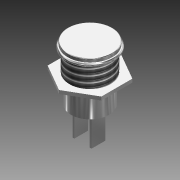
# Autodesk Inventor part: Hohlstecker
Saved by Autodesk Inventor 2013 SP1 (Build 170176100, 176)
## iProperties
Created: 2012-12-09
Part Number: Hohlstecker
Material: Stahl, verchromt
Document SubType Name: Modeling
Designer: Sebastian
Density: 1 g/cm^3
Author: Sebastian
Autodesk Inventor part; units mm, degrees
note: some values were not read from the file. Chosen so that the rebuilt part matches the saved one: edges of "Rundung1".
ref_plane "YZ Plane" through (0, 0, 0) normal (1, 0, 0) x (0, 1, 0)
ref_plane "XZ Plane" through (0, 0, 0) normal (0, 1, 0) x (-1, 0, 0)
ref_plane "XY Plane" through (0, 0, 0) normal (0, 0, 1) x (1, 0, 0)
sketch "Skizze1" plane through (0, 0, 0) normal (0, 0, 1) x (1, 0, 0)
  circle A0 centre (0, 0) radius 5.5
  dimension "d0" = 11
  constraints: 1 centre point, 1 coincident
  measures "d0" diameter of A0
extrude "Extrusion1" add sketch "Skizze1" against normal blind 6
sketch "Skizze2" plane through (0, 0, 0) normal (0, 0, 1) x (1, 0, 0)
  circle A0 centre (0, 0) radius 6
  dimension "d5" = 12
  constraints: 1 centre point, 1 coincident
  measures "d5" diameter of A0
extrude "Extrusion2" add sketch "Skizze2" along normal blind 8 separate body
thread "Gewinde1" size "M12x1.75" class "6g" standard "ANSI Metric M Profile" full length
sketch "Skizze3" plane through (0, 0, 0) normal (0, 0, 1) x (1, 0, 0)
  circle A0 centre (0, 0) radius 5.75
  dimension "d10" = 11.5
  constraints: 1 centre point, 1 coincident
  measures "d10" diameter of A0
extrude "Extrusion3" add sketch "Skizze3" along normal blind 1 separate body
move or copy body "Körper verschieben1" bodies to move or copy 3 copy no translate (0, 0, 8)
fillet "Rundung1" radius 0.5 1 edges at (-6, 0, 0)
sketch "Skizze4" plane through (0, 0, 0) normal (0, 0, 1) x (1, 0, 0)
  circle A0 centre (0, 0) radius 6.5
  dimension "d19" = 13
  constraints: 1 centre point, 1 coincident
  measures "d19" diameter of A0
extrude "Extrusion4" add sketch "Skizze4" along normal blind 1 separate body
move or copy body "Körper verschieben2" bodies to move or copy 4 copy no translate (0, 0, 9)
fillet "Rundung2" radius 0.25 1 edges at (-6.5, 0, 10)
sketch "Skizze5" plane through (0, 0, 0) normal (0, 1, 0) x (-1, 0, 0)
  circle A0 centre (6.5, 0) radius 0.5
  line L0 (0, -3.25) -> (0, 3.25)
  line L1 (0, 0) -> (6.5, 0) construction
  dimension "d26" = 1
  dimension "d27" = 6.5
  constraints: 4 end point, 1 centre point, 1 horizontal, 1 perpendicular
  measures "d26" diameter of A0
  measures "d27" distance of L1.start L1.end
revolve "Umdrehung1" add sketch "Skizze5" angle 360 about axis through (0, 0, -3.25) along (0, 0, 1) separate body
move or copy body "Körper verschieben3" bodies to move or copy 5 copy no translate (0, 0, 8.5)
sketch "Skizze6" plane through (0, 0, 0) normal (0, 0, 1) x (1, 0, 0)
  line L0 (0, 9) -> (7.7942, 4.5)
  line L1 (7.7942, 4.5) -> (7.7942, -4.5)
  line L2 (7.7942, -4.5) -> (0, -9)
  line L3 (0, -9) -> (-7.7942, -4.5)
  line L4 (-7.7942, -4.5) -> (-7.7942, 4.5)
  line L5 (-7.7942, 4.5) -> (0, 9)
  circle A0 centre (0, 0) radius 6
  dimension "d32" = 12
  constraints: 12 end point, 2 coincident, 1 centre point, 13 other
  measures "d32" diameter of A0
extrude "Extrusion5" add sketch "Skizze6" along normal blind 1 separate body
move or copy body "Körper verschieben4" bodies to move or copy 6 copy no translate (0, 0, 1)
sketch "Skizze7" plane through (0, 0, 0) normal (0, 0, 1) x (1, 0, 0)
  line L0 (-3.066, -2) -> (-2.566, -2)
  line L1 (-2.566, -2) -> (-2.566, 2)
  line L2 (-2.566, 2) -> (-3.066, 2)
  line L3 (-3.066, 2) -> (-3.066, -2)
  line L4 (-3.066, -2) -> (-2.566, 2) construction
  line L5 (-2.566, -2) -> (-3.066, 2) construction
  line L6 (1.9662, -2.029) -> (2.4662, -2.029)
  line L7 (2.4662, -2.029) -> (2.4662, 1.971)
  line L8 (2.4662, 1.971) -> (1.9662, 1.971)
  line L9 (1.9662, 1.971) -> (1.9662, -2.029)
  line L10 (1.9662, -2.029) -> (2.4662, 1.971) construction
  line L11 (2.4662, -2.029) -> (1.9662, 1.971) construction
  point P0 (0, 0)
  point P1 (-2.816, 0)
  point P2 (2.2162, -0.029)
  dimension "d38" = 0.5
  dimension "d39" = 4
  dimension "d40" = 0.5
  dimension "d41" = 4
  constraints: 24 end point, 4 midpoint, 4 parallel, 2 horizontal, 2 perpendicular
  measures "d38" distance of L2.end L1.end
  measures "d39" distance of L1.end L0.end
  measures "d40" distance of L8.end L7.end
  measures "d41" distance of L7.end L6.end
extrude "Extrusion6" add sketch "Skizze7" against normal blind 9 separate body
move or copy body "Körper verschieben5" bodies to move or copy 7 copy no translate (0, 0, -6)
